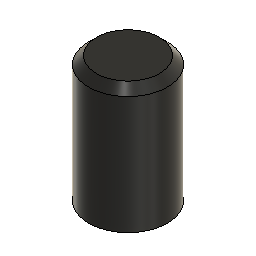
Pin (Autodesk Fusion 360 design; units mm, degrees)
part number: 2026-05-27-02-31-01-321
Autodesk Fusion 360 part; units mm, degrees
sketch "Sketch1" plane through (0, 0, 0) normal (0, 0, 1) x (1, 0, 0)
  circle A0 centre (40, 25) radius 2.5
  dimension "d1" = 5
  measures "d1" diameter of A0
extrude "Extrude1" add sketch "Sketch1" along normal blind 8
chamfer "Chamfer1" distance 0.5 angle 45 1 edges at (37.6692, 24.096, 8)
